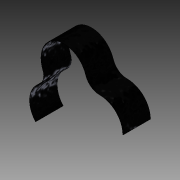
# Autodesk Inventor part: Sheild
Saved by Autodesk Inventor 2013 (Build 170138000, 138)
## iProperties
Created: 2013-06-27
Part Number: Sheild
Material: Generic
Document SubType Name: Modeling
Designer: mvarma
Density: 1 g/cm^3
Author: mvarma
Autodesk Inventor part; units mm, degrees
ref_plane "YZ Plane" through (0, 0, 0) normal (1, 0, 0) x (0, 1, 0)
ref_plane "XZ Plane" through (0, 0, 0) normal (0, 1, 0) x (-1, 0, 0)
ref_plane "XY Plane" through (0, 0, 0) normal (0, 0, 1) x (1, 0, 0)
sketch "Sketch1" plane through (0, 0, 0) normal (0, 0, 1) x (1, 0, 0)
  arc A0 (67.8806, 113.5366) -> (74.024, 136.5789) centre (56.3452, 128.9522) ccw
  line L0 (63.0849, 61.9574) -> (112.0151, 5.0878) construction
  arc A1 (67.8806, 113.5366) -> (63.0849, 61.9574) centre (88.8014, 85.5789) ccw
  arc A2 (139.2877, 161.4802) -> (160.6194, 146.2689) centre (160.3908, 168.5113) ccw
  arc A3 (170.156, 145.0434) -> (160.6194, 146.2689) centre (160.9785, 111.3458) ccw
  line L1 (195.9029, 111.1496) -> (195.4212, 25.3733) construction
  ellipse E0 centre (106.1636, 150.4439) end of major axis (106.1759, 186.8392) minor radius 34.7604 (139.2877, 161.4802) -> (74.024, 136.5789) ccw
  arc A4 (112.0151, 5.0878) -> (112.3757, 4.7043) centre (116.5302, 8.9726) ccw
  arc A5 (112.3757, 4.7043) -> (195.1395, 23.7862) centre (147.6111, 40.9044) ccw construction
  arc A6 (195.1395, 23.7862) -> (195.4212, 25.3733) centre (190.6588, 25.4) ccw construction
  arc A7 (195.9029, 111.1496) -> (170.156, 145.0434) centre (160.9785, 111.3458) ccw
  arc A8 (67.4051, 114.1722) -> (73.2902, 136.2761) centre (56.3452, 128.9522) ccw
  arc A9 (67.4051, 114.1722) -> (62.4916, 61.4299) centre (88.8014, 85.5789) ccw
  line L2 (62.4916, 61.4299) -> (111.4134, 4.5701) construction
  arc A10 (111.4134, 4.5701) -> (111.8221, 4.1355) centre (116.5302, 8.9726) ccw construction
  arc A11 (111.8221, 4.1355) -> (195.8863, 23.5172) centre (147.6111, 40.9044) ccw construction
  arc A12 (195.8863, 23.5172) -> (196.2149, 25.3688) centre (190.6588, 25.4) ccw construction
  line L3 (196.2149, 25.3688) -> (196.6967, 111.1452) construction
  arc A13 (196.6967, 111.1452) -> (170.3646, 145.8092) centre (160.9785, 111.3458) ccw
  arc A14 (170.3646, 145.8092) -> (160.6113, 147.0626) centre (160.9785, 111.3458) ccw
  arc A15 (140.0441, 161.7212) -> (160.6113, 147.0626) centre (160.3908, 168.5113) ccw
  line L4 (62.4916, 61.4299) -> (63.0849, 61.9574)
  line L5 (195.9029, 111.1496) -> (196.6967, 111.1452)
  spline S0 degree 5 poles (140.0441, 161.7212) (139.583, 163.2368) (139.0439, 164.7287) (138.4279, 166.1913) (135.5266, 172.185) (131.3399, 177.4697) (127.4753, 180.9092) (118.7418, 186.2077) (108.7095, 188.0956) (103.6086, 188.0948) (93.5768, 186.2035) (84.8447, 180.9023) (80.981, 177.4616) (74.5342, 169.3198) (71.1378, 159.497) (70.2772, 154.2953) (70.2947, 147.4301) (71.7711, 140.8127) (72.1989, 139.2737) (72.7058, 137.7596) (73.2902, 136.2761) knots 0 0 0 0 0 0 0.067503 0.067503 0.067503 0.283346 0.283346 0.283346 0.495621 0.495621 0.495621 0.711472 0.711472 0.711472 0.932057 0.932057 0.932057 1 1 1 1 1 1
  point P0 (0, 0)
  point P1 (93.6139, 184.384)
  point P2 (71.7596, 145.2447)
  point P3 (61.2825, 107.0736)
  point P4 (135.0639, 170.6681)
  point P5 (195.5971, 56.6944)
  point P6 (88.1705, 44.9716)
  dimension "d27" = 0.7937
  constraints: 33 point on circle, 16 centre point, 12 end point, 2 coincident, 2 tangent, 1 concentric, 1 perpendicular, 1 point on line, 57 other
  measures "d27" radial gap between concentric circles of A1 A9
extrude "Extrusion1" add sketch "Sketch1" along normal blind 42.164
body "Solid1"
